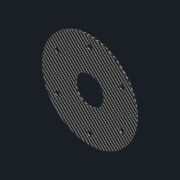
# Autodesk Inventor part: unit-plate1
Saved by Autodesk Inventor 2021 (Build 250183000, 183)
## iProperties
Created: 2021-07-12
Part Number: unit-plate1
Material: CFRP
Document SubType Name: Sheet Metal
Designer: yuta0
Density: 1.43 g/cm^3
Sheet Metal Rule: Default_mm
Appearance: カーボンファイバー
Author: yuta0
Autodesk Inventor part; units mm, degrees
ref_plane "YZ Plane" through (0, 0, 0) normal (1, 0, 0) x (0, 1, 0)
ref_plane "XZ Plane" through (0, 0, 0) normal (0, 1, 0) x (-1, 0, 0)
ref_plane "XY Plane" through (0, 0, 0) normal (0, 0, 1) x (1, 0, 0)
sketch "スケッチ1" plane through (0, 0, 0) normal (0, 0, 1) x (1, 0, 0)
  circle A0 centre (0, 0) radius 40.5
  dimension "d0" = 81
  measures "d0" diameter of A0
extrude "プレート1" add sketch "スケッチ1" along normal mid plane 1
sketch "スケッチ2" plane through (0, 0, 0.5) normal (0, 0, 1) x (1, 0, 0)
  circle A0 centre (0, 0) radius 12
  dimension "d2" = 24
  constraints: 1 centre point, 1 coincident
  measures "d2" diameter of A0
extrude "押し出し1" cut sketch "スケッチ2" against normal blind 10
sketch "スケッチ3" plane through (0, 0, 0.5) normal (0, 0, 1) x (1, 0, 0)
  circle A0 centre (0, 0) radius 32
  point P0 (0, 32)
  point P1 (-27.7128, 16)
  point P2 (-27.7128, -16)
  point P3 (0, -32)
  point P4 (27.7128, -16)
  point P5 (27.7128, 16)
  dimension "d5" = 64
  dimension "d8" = 360
  constraints: 1 coincident, 1 vertical alignment, 9 other
hole "穴1" at (0, 32, 0.5) at (-27.7128, 16, 0.5) at (-27.7128, -16, 0.5) at (0, -32, 0.5) at (27.7128, -16, 0.5) at (27.7128, 16, 0.5) direction (0, 0, -1) diameter 4.5 end through all clearance for "Flat Head Machine Screw" size "M4" standard "Ansi Metric M Profile"
equation "\"d15\" = Thickness"
equation "\"d1\" = Thickness"
equation "\"BendRadius\" = Thickness"
equation "\"BendReliefWidth\" = Thickness"
equation "\"BendReliefDepth\" = 0.5 * Thickness"
equation "\"CornerReliefSize\" = 4 * Thickness"
equation "\"MinimumRemnant\" = 2 * Thickness"
equation "\"TransitionRadius\" = BendRadius"
equation "\"JacobiRadiusSize\" = BendRadius"
equation "\"GapSize\" = Thickness"
equation "\"Thickness\" = 1"
